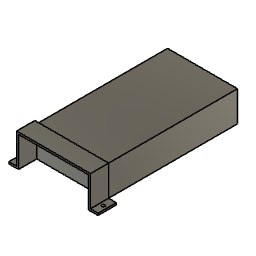
PSU_Mounting (Autodesk Fusion 360 design; units mm, degrees)
Autodesk Fusion 360 part; units mm, degrees
sketch "Sketch1" plane through (0, 0, 0) normal (0, 0, 1) x (1, 0, 0) in component "PSU"
  line L0 (-40.64, 66.04) -> (74.36, 66.04)
  line L1 (74.36, 66.04) -> (74.36, -148.96)
  line L2 (74.36, -148.96) -> (-40.64, -148.96)
  line L3 (-40.64, -148.96) -> (-40.64, 66.04)
  dimension "d1" = 115
  dimension "d2" = 215
  constraint horizontal L0
  constraint vertical L1
  constraint horizontal L2
  constraint vertical L3
  measures "d1" distance of L0.start L0.end
  measures "d2" distance of L0.end L1.end
extrude "Extrude1" add sketch "Sketch1" along normal blind 50 makes body 1 in component "PSU"
sketch "Sketch1 (2)" plane through (0, -148.96, 0) normal (0, -1, 0) x (1, 0, 0) in component "Bracket"
  line L0 (-40.64, 0) -> (74.36, 0)
  line L1 (74.36, 0) -> (74.36, 50)
  line L2 (74.36, 50) -> (-40.64, 50)
  line L3 (-40.64, 50) -> (-40.64, 0)
  line L4 (-56.515, 0) -> (-40.64, 0)
  line L5 (-40.64, 50) -> (74.36, 50)
  line L6 (74.36, 0) -> (90.235, 0)
  line L7 (90.235, 0) -> (90.235, 3.175)
  line L8 (90.235, 3.175) -> (77.535, 3.175)
  line L9 (77.535, 3.175) -> (77.535, 53.175)
  line L10 (77.535, 53.175) -> (-43.815, 53.175)
  line L11 (-43.815, 53.175) -> (-43.815, 3.175)
  line L12 (-43.815, 3.175) -> (-56.515, 3.175)
  line L13 (-56.515, 3.175) -> (-56.515, 0)
  dimension "d5" = 3.175
  dimension "d6" = 3.175
  dimension "d7" = 12.7
  dimension "d8" = 3.175
  dimension "d9" = 3.175
  dimension "d10" = 3.175
  dimension "d11" = 12.7
  constraint coincident L0.start L3.end
  constraint perpendicular L3 L4
  constraint coincident L2.end L3.start
  constraint coincident L1.end L2.start
  constraint coincident L0.end L1.start
  constraint perpendicular L1 L6
  constraint perpendicular L0 L7
  constraint perpendicular L7 L8
  constraint perpendicular L8 L9
  constraint perpendicular L9 L10
  constraint perpendicular L10 L11
  constraint perpendicular L11 L12
  constraint perpendicular L12 L13
  measures "d5" distance of L4.start L12.end
  measures "d6" distance of L3 L11
  measures "d7" distance of L11.end L12.end
  measures "d8" distance of L5 L10
  measures "d9" distance of L1 L9
  measures "d10" distance of L6 L8
  measures "d11" distance of L7.end L8.end
extrude "Extrude1'" add sketch "Sketch1 (2)" along normal blind 30 separate body contours L1 L2 L3 L4 L5 L6 L7 L8 L9 L10 L11 L12 L13 makes body 2 in component "Bracket"
sketch "Sketch2" plane through (0, 0, 3.175) normal (0, 0, 1) x (-1, 0, 0) in component "Bracket"
  line L0 (43.815, 148.96) -> (56.515, 148.96)
  line L1 (56.515, 148.96) -> (56.515, 178.96)
  line L2 (56.515, 178.96) -> (43.815, 178.96)
  line L3 (43.815, 178.96) -> (43.815, 148.96)
  circle A0 centre (50.165, 163.96) radius 2.5
  circle A1 centre (-83.885, 163.96) radius 2.5
  line L4 (-90.235, 148.96) -> (-90.235, 178.96)
  line L5 (-90.235, 148.96) -> (-77.535, 148.96)
  dimension "d14" = 5
  dimension "d15" = 15
  dimension "d16" = 6.35
  dimension "d17" = 6.35
  dimension "d18" = 15
  dimension "d19" = 5
  measures "d14" diameter of A0
  measures "d15" distance of L0 A0.centre
  measures "d16" distance of L1 A0.centre
  measures "d17" distance of A1.centre L4
  measures "d18" distance of A1.centre L5
  measures "d19" diameter of A1
extrude "Extrude1''" cut sketch "Sketch2" against normal through all contours A0 | A1 bodies 2 in component "Bracket"
component "PSU" placed x (1, 0, 0) y (0, 1, 0) z (0, 0, 1) at (0, 0, 0)
component "Bracket" placed x (1, 0, 0) y (0, 1, 0) z (0, 0, 1) at (0, 0, 0)
